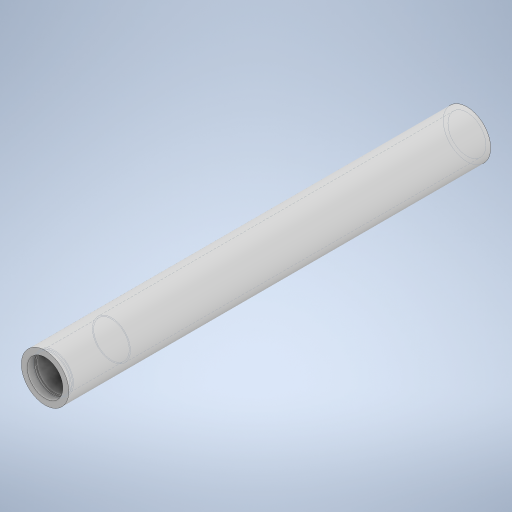
# Autodesk Inventor part: body
Saved by Autodesk Inventor 2023 (Build 270158000, 158)
## iProperties
Created: 2023-07-16
Part Number: body
Material: Generic
Document SubType Name: Modeling
Designer: checo
Density: 1 g/cm^3
Appearance: Default
Author: checo
Autodesk Inventor part; units mm, degrees
ref_plane "YZ Plane" through (0, 0, 0) normal (1, 0, 0) x (0, 1, 0)
ref_plane "XZ Plane" through (0, 0, 0) normal (0, 1, 0) x (-1, 0, 0)
ref_plane "XY Plane" through (0, 0, 0) normal (0, 0, 1) x (1, 0, 0)
sketch "Sketch1" plane through (0, 0, 0) normal (0, 0, 1) x (1, 0, 0)
  circle A0 centre (0, 0) radius 7.5
  circle A1 centre (0, 0) radius 10
  dimension "d0" = 15
  dimension "d1" = 20
  constraints: 2 centre point, 2 coincident
  measures "d0" diameter of A0
  measures "d1" diameter of A1
extrude "Extrusion1" add sketch "Sketch1" along normal blind 24
sketch "Sketch2" plane through (0, 0, 0) normal (0, 0, -1) x (-1, 0, 0)
  circle A0 centre (0, 0) radius 8
  circle A1 centre (0, 0) radius 7.5 projected
  circle A2 centre (0, 0) radius 10 projected
  circle A3 centre (0, 0) radius 7.5 projected
  circle A4 centre (0, 0) radius 10 projected
  circle A5 centre (0, 0) radius 7.5 projected
  circle A6 centre (0, 0) radius 10 projected
  circle A7 centre (0, 0) radius 7.5 projected
  dimension "d4" = 16
  constraints: 1 centre point, 1 coincident
  measures "d4" diameter of A0
extrude "Extrusion2" add sketch "Sketch2" along normal blind 150 contours A2
sketch "Sketch3" plane through (0, 0, 24) normal (0, 0, 1) x (1, 0, 0)
  circle A0 centre (0, 0) radius 10 projected
  circle A1 centre (0, 0) radius 7.5 projected
  circle A2 centre (0, 0) radius 8
  dimension "d7" = 0.5
  constraints: 1 centre point, 1 coincident
  measures "d7" radial gap between concentric circles of A1 A2
extrude "Extrusion3" add sketch "Sketch3" along normal blind 1 contours A0
sketch "Sketch4" plane through (0, 0, 25) normal (0, 0, 1) x (1, 0, 0)
  circle A0 centre (0, 0) radius 10 projected
  circle A1 centre (0, 0) radius 7.5 projected
extrude "Extrusion4" add sketch "Sketch4" along normal blind 3
body "Solid1"
